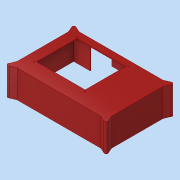
# Autodesk Inventor part: vna_cover
Saved by Autodesk Inventor 2022 (Build 260153000, 153)
## iProperties
Created: 2020-10-01
Part Number: vna_cover
Material: Generic
Document SubType Name: Modeling
Designer: nnico
Density: 1 g/cm^3
Appearance: Red
Author: nnico
Autodesk Inventor part; units mm, degrees
ref_plane "YZ Plane" through (0, 0, 0) normal (1, 0, 0) x (0, 1, 0)
ref_plane "XZ Plane" through (0, 0, 0) normal (0, 1, 0) x (-1, 0, 0)
ref_plane "XY Plane" through (0, 0, 0) normal (0, 0, 1) x (1, 0, 0)
sketch "Sketch1" plane through (0, 0, 0) normal (0, 1, 0) x (-1, 0, 0)
  line L0 (175, -115) -> (-175, -115)
  line L1 (-175, -115) -> (-175, 115)
  line L2 (-175, 115) -> (175, 115)
  line L3 (175, 115) -> (175, -115)
  line L4 (0, -115) -> (0, 115) construction
  line L5 (175, 0) -> (-175, 0) construction
  point P0 (0, 0)
  point P1 (0, 0)
  dimension "d0" = 350
  dimension "d1" = 230
  constraints: 12 end point, 5 midpoint, 2 parallel, 1 coincident, 1 horizontal, 1 perpendicular
  measures "d0" distance of L1.end L2.end
  measures "d1" distance of L0.end L1.end
extrude "Extrusion1" add sketch "Sketch1" along normal blind 3
sketch "Sketch6" plane through (0, 3, 0) normal (0, 1, 0) x (1, 0, 0)
  line L0 (175, 115) -> (-175, 115) construction
  line L1 (0, 115) -> (0, -115) construction
  line L2 (175, -115) -> (-175, -115) construction
  line L3 (-175, 115) -> (-175, -115) construction
  line L4 (-175, 0) -> (175, 0) construction
  line L5 (175, -115) -> (175, 115) construction
  circle A0 centre (-179, 119) radius 6
  line L6 (-175, 115) -> (-179, 115) construction
  line L7 (-179, 115) -> (-179, 119) construction
  line L8 (-179, 119) -> (-175, 119) construction
  line L9 (-175, 119) -> (-175, 115) construction
  line L10 (-155, 115) -> (-175.4528, 123.8392)
  line L11 (-175, 95) -> (-183.0203, 114.5461)
  line L12 (-175, 95) -> (-175, 115)
  line L13 (-155, 115) -> (-175, 115)
  circle A1 centre (-179, -119) radius 6
  line L14 (-155, -115) -> (-175.4528, -123.8392)
  line L15 (-175, -95) -> (-183.0203, -114.5461)
  line L16 (-175, -95) -> (-175, -115)
  line L17 (-155, -115) -> (-175, -115)
  circle A2 centre (179, 119) radius 6
  line L18 (155, 115) -> (175.4528, 123.8392)
  line L19 (175, 95) -> (183.0203, 114.5461)
  line L20 (175, 95) -> (175, 115)
  line L21 (155, 115) -> (175, 115)
  line L22 (175, -95) -> (183.0203, -114.5461)
  circle A3 centre (179, -119) radius 6
  line L23 (155, -115) -> (175.4528, -123.8392)
  line L24 (155, -115) -> (175, -115)
  line L25 (175, -95) -> (175, -115)
  circle A4 centre (179, -119) radius 2.75
  circle A5 centre (179, 119) radius 2.75
  circle A6 centre (-179, -119) radius 2.75
  circle A7 centre (-179, 119) radius 2.75
  point P0 (0, 0)
  dimension "d22" = 12
  dimension "d23" = 4
  dimension "d24" = 4
  dimension "d25" = 20
  dimension "d26" = 20
  dimension "d30" = 5.5
  constraints: 44 end point, 17 symmetric about line, 8 centre point, 8 point on circle, 4 midpoint, 2 coincident, 2 collinear, 2 parallel, 2 point on line, 1 horizontal, 1 perpendicular, 6 other
  measures "d22" diameter of A0
  measures "d23" distance of L7.end L8.end
  measures "d24" distance of L6.end L7.end
  measures "d25" distance of L10.start L0.end
  measures "d26" distance of L11.start L0.end
  measures "d30" diameter of A4
extrude "Extrusion6" add sketch "Sketch6" against normal blind 103 contours A0 L13 L12 | A0 L10 L13 | A0 L12 L11 | A1 L16 L17 | L15 L16 A1 | A1 L17 L14 | A2 L20 L21 | A2 L21 L18 | L19 L20 A2 | L22 A3 L25 | A3 L24 L25 | A3 L23 L24 | A4 | A5 | A6 | A7 picked at (-175.087, 116.3056) picked at (-175.087, -116.3056) picked at (175.0917, 116.2969) picked at (175.0917, -116.2969)
sketch "Sketch9" plane through (0, 0, 0) normal (0, -1, 0) x (1, 0, 0)
  line L0 (-175, -95) -> (-175, -115) projected
  line L1 (175, 115) -> (175, 95) projected
  line L2 (-175, -115) -> (175, -115)
  line L3 (175, -115) -> (175, 115)
  line L4 (175, 115) -> (-175, 115)
  line L5 (-175, 115) -> (-175, -115)
  line L6 (-173, -113) -> (173, -113)
  line L7 (173, -113) -> (173, 113)
  line L8 (173, 113) -> (-173, 113)
  line L9 (-173, 113) -> (-173, -113)
  line L10 (0, -115) -> (0, 115) construction
  line L11 (-155, 115) -> (155, 115) construction
  point P0 (0, 0)
  dimension "d31" = 2
  dimension "d32" = 2
  dimension "d33" = 2
  dimension "d34" = 2
  constraints: 18 end point, 4 parallel, 2 horizontal, 2 midpoint, 2 perpendicular
  measures "d31" distance between parallel lines of L5 L9
  measures "d32" distance between parallel lines of L7 L3
  measures "d33" distance between parallel lines of L4 L8
  measures "d34" distance between parallel lines of L2 L6
extrude "Extrusion7" add sketch "Sketch9" along normal blind 100
sketch "Sketch10" plane through (155, 3, -115) normal (0, 0, -1) x (-1, 0, 0)
  line L0 (0, -103) -> (310, -103) projected
  line L1 (17, -103) -> (267, -103)
  line L2 (267, -103) -> (267, -48)
  line L3 (267, -48) -> (17, -48)
  line L4 (17, -48) -> (17, -103)
  line L5 (0, 0) -> (0, -103) projected
  line L6 (310, 0) -> (0, 0) construction
  line L7 (155, 0) -> (155, -103) construction
  line L8 (267, -48) -> (187, -48)
  line L9 (187, -48) -> (187, -23)
  line L10 (187, -23) -> (267, -23)
  line L11 (267, -23) -> (267, -48)
  point P0 (155, -3)
  point P1 (-18, -103)
  dimension "d38" = 55
  dimension "d39" = 35
  dimension "d40" = 250
  dimension "d41" = 25
  dimension "d42" = 80
  constraints: 18 end point, 4 parallel, 3 perpendicular, 2 horizontal, 2 point on line, 1 midpoint
  measures "d38" distance of L1.end L2.end
  measures "d39" distance from line of point (-18, -103) L4
  measures "d40" distance of L2.end L3.end
  measures "d41" distance of L8.end L9.end
  measures "d42" distance of L9.end L10.end
extrude "Extrusion8" cut sketch "Sketch10" against normal up to next
sketch "Sketch11" plane through (0, 3, 0) normal (0, 1, 0) x (1, 0, 0)
  line L0 (-138, 90) -> (42, 90)
  line L1 (42, 90) -> (42, -60)
  line L2 (42, -60) -> (-138, -60)
  line L3 (-138, -60) -> (-138, 90)
  line L4 (-173, -113) -> (-173, 113) projected
  line L5 (-173, 113) -> (173, 113) projected
  point P0 (0, 0)
  dimension "d45" = 180
  dimension "d46" = 150
  dimension "d47" = 35
  dimension "d48" = 173
  constraints: 8 end point, 2 parallel, 1 horizontal, 1 perpendicular
  measures "d45" distance of L1.end L2.end
  measures "d46" distance of L0.end L1.end
  measures "d47" distance between parallel lines of L4 L3
  measures "d48" distance between parallel lines of L5 L2
extrude "Extrusion9" cut sketch "Sketch11" against normal up to next
sketch "Sketch13" plane through (0, -100, 0) normal (0, -1, 0) x (1, 0, 0)
  arc A0 (-183.0203, -114.5461) -> (-175.4528, -123.8392) centre (-179, -119) ccw projected
  line L0 (-175, 95) -> (-175, -95) construction
  line L1 (-175, 0) -> (175, 0) construction
  line L2 (175, 95) -> (175, -95) construction
  line L3 (155, -115) -> (-155, -115) construction
  line L4 (0, -115) -> (0, 115) construction
  line L5 (-155, 115) -> (155, 115) construction
  circle A1 centre (-179, 119) radius 2.75
  circle A2 centre (179, 119) radius 2.75
  circle A3 centre (-179, -119) radius 2.75
  circle A4 centre (179, -119) radius 2.75
  point P0 (0, 0)
  dimension "d51" = 5.5
  constraints: 9 symmetric about line, 4 centre point, 4 end point, 4 midpoint, 3 coincident, 3 other
  measures "d51" diameter of A1
extrude "Extrusion10" cut sketch "Sketch13" against normal blind 7
sketch "Sketch14" plane through (0, 3, 0) normal (0, 1, 0) x (1, 0, 0)
  line L0 (-138, 90) -> (42, 90) construction
  line L1 (-138, -60) -> (-138, 90) construction
  line L2 (42, -60) -> (-138, -60) construction
  line L3 (42, 90) -> (42, -60) construction
  line L4 (-143, 95) -> (47, 95) construction
  line L5 (47, 95) -> (47, -65) construction
  line L6 (47, -65) -> (-143, -65) construction
  line L7 (-143, -65) -> (-143, 95) construction
  circle A0 centre (-143, 95) radius 3
  circle A1 centre (-143, 95) radius 1.75
  line L8 (-48, 95) -> (-48, -65) construction
  line L9 (-143, 15) -> (47, 15) construction
  circle A2 centre (47, 95) radius 3
  circle A3 centre (47, 95) radius 1.75
  circle A4 centre (-143, -65) radius 3
  circle A5 centre (-143, -65) radius 1.75
  circle A6 centre (47, -65) radius 3
  circle A7 centre (47, -65) radius 1.75
  point P0 (0, 0)
  dimension "d54" = 5
  dimension "d55" = 5
  dimension "d56" = 5
  dimension "d57" = 5
  dimension "d58" = 6
  dimension "d59" = 3.5
  constraints: 12 end point, 8 centre point, 6 symmetric about line, 5 coincident, 4 midpoint, 2 parallel, 1 horizontal, 1 perpendicular, 6 other
  measures "d54" distance between parallel lines of L5 L3
  measures "d55" distance between parallel lines of L4 L0
  measures "d56" distance between parallel lines of L7 L1
  measures "d57" distance between parallel lines of L2 L6
  measures "d58" diameter of A0
  measures "d59" diameter of A1
extrude "Extrusion11" cut sketch "Sketch14" against normal up to next contours A1 | A3 | A5 | A7
sketch "Sketch15" plane through (0, 3, 0) normal (0, 1, 0) x (1, 0, 0)
  circle A0 centre (47, 95) radius 1.75 projected
  circle A1 centre (47, 95) radius 3.25
  line L0 (-138, 90) -> (42, 90) construction
  line L1 (42, 90) -> (42, -60) construction
  line L2 (42, -60) -> (-138, -60) construction
  line L3 (-138, -60) -> (-138, 90) construction
  line L4 (42, -60) -> (42, 90) construction
  line L5 (42, 15) -> (-138, 15) construction
  line L6 (-138, 90) -> (-138, -60) construction
  line L7 (42, 90) -> (-138, 90) construction
  line L8 (-48, 90) -> (-48, -60) construction
  circle A2 centre (47, -65) radius 3.25
  circle A3 centre (-143, 95) radius 3.25
  circle A4 centre (-143, -65) radius 3.25
  circle A5 centre (47, -65) radius 1.75 projected
  circle A6 centre (-143, -65) radius 1.75 projected
  circle A7 centre (-143, 95) radius 1.75 projected
  point P0 (0, 0)
  dimension "d62" = 6.5
  constraints: 4 centre point, 4 end point, 4 midpoint, 3 symmetric about line, 1 coincident, 3 other
  measures "d62" diameter of A1
extrude "Extrusion12" add sketch "Sketch15" against normal blind 4
body "Solid1"
